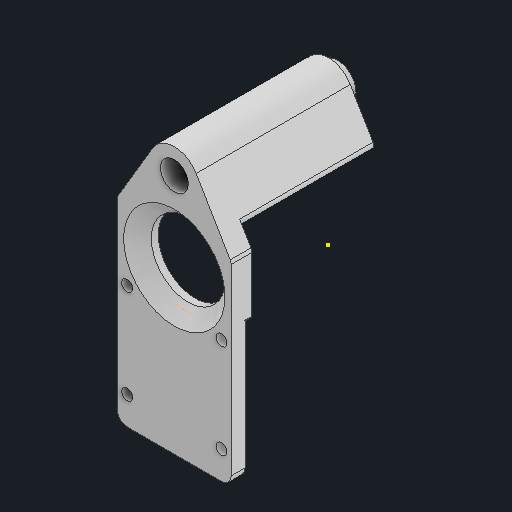
# Autodesk Inventor part: servo_side_plate1
Saved by Autodesk Inventor 2026 (Build 300175000, 175)
## iProperties
Created: 2025-12-05
Part Number: servo_side_plate1
Material: Generic
Document SubType Name: Modeling
Designer: numai
Density: 1 g/cm^3
Appearance: Default
Author: numai
Autodesk Inventor part; units mm, degrees
ref_plane "YZ Plane" through (0, 0, 0) normal (1, 0, 0) x (0, 1, 0)
ref_plane "XZ Plane" through (0, 0, 0) normal (0, 1, 0) x (-1, 0, 0)
ref_plane "XY Plane" through (0, 0, 0) normal (0, 0, 1) x (1, 0, 0)
ref_plane "作業平面1" through (0, -9.5185, 2.5) normal (0, 0, 1) x (1, 0, 0)
sketch "スケッチ1" plane through (0, -9.5185, 2.5) normal (0, 0, 1) x (1, 0, 0)
  arc A0 (6.111, 12.2244) -> (9.9756, 16.2085) centre (0, 22.0185) ccw construction
  arc A1 (7, 11.2305) -> (6.111, 12.2244) centre (6, 11.2305) ccw construction
  line L0 (7, 11.2305) -> (7, -12.0915) construction
  arc A2 (6.6057, -12.8872) -> (7, -12.0915) centre (6, -12.0915) ccw construction
  arc A3 (6.6057, -12.8872) -> (7.8, -11.5915) centre (6.5, -11.5915) ccw construction
  line L1 (7.8, -10.5915) -> (7.8, -11.5915) construction
  arc A4 (10.11, -8.2815) -> (7.8, -10.5915) centre (10.11, -10.5915) ccw construction
  line L2 (10.86, -8.2815) -> (10.11, -8.2815) construction
  arc A5 (10.86, -8.2815) -> (12.16, -6.9815) centre (10.86, -6.9815) ccw construction
  line L3 (12.16, 16.2085) -> (12.16, -6.9815) construction
  line L4 (9.9756, 16.2085) -> (12.16, 16.2085) construction
  circle A6 centre (10.25, 13.5185) radius 0.7835 construction
  circle A7 centre (10.25, -6.9815) radius 0.7835 construction
  arc A8 (-7.8, -11.5915) -> (-6.6057, -12.8872) centre (-6.5, -11.5915) ccw construction
  arc A9 (-7, -12.0915) -> (-6.6057, -12.8872) centre (-6, -12.0915) ccw construction
  line L5 (-7, -12.0915) -> (-7, 11.2305) construction
  arc A10 (-6.111, 12.2244) -> (-7, 11.2305) centre (-6, 11.2305) ccw construction
  arc A11 (-9.9756, 16.2085) -> (-6.111, 12.2244) centre (0, 22.0185) ccw construction
  line L6 (-12.16, 16.2085) -> (-9.9756, 16.2085) construction
  line L7 (-12.16, -6.9815) -> (-12.16, 16.2085) construction
  arc A12 (-12.16, -6.9815) -> (-10.86, -8.2815) centre (-10.86, -6.9815) ccw construction
  line L8 (-10.11, -8.2815) -> (-10.86, -8.2815) construction
  arc A13 (-7.8, -10.5915) -> (-10.11, -8.2815) centre (-10.11, -10.5915) ccw construction
  line L9 (-7.8, -11.5915) -> (-7.8, -10.5915) construction
  circle A14 centre (-10.25, 13.5185) radius 0.7835 construction
  circle A15 centre (-10.25, -6.9815) radius 0.7835 construction
  line L10 (-12.36, 16.2085) -> (-12.36, -6.9815) construction
  line L11 (12.36, -6.9815) -> (12.36, 16.2085) construction
  circle A16 centre (0, 22.0185) radius 3.4 construction
  arc A17 (5.25, 16.6624) -> (-5.25, 16.6624) centre (0, 22.0185) ccw construction
  arc A18 (-5.25, 16.6624) -> (5.25, 16.6624) centre (0, 22.0185) ccw construction
  circle A19 centre (0, 22.0185) radius 8
  arc A20 (10.25, -13.0915) -> (12.36, -10.9815) centre (10.25, -10.9815) ccw construction
  arc A21 (-12.36, -10.9815) -> (-10.25, -13.0915) centre (-10.25, -10.9815) ccw construction
  arc A22 (-11.9207, 29.8679) -> (-12.36, 28.8072) centre (-10.86, 28.8072) ccw projected
  line L12 (-10.0993, 31.6892) -> (-11.9207, 29.8679) projected
  arc A23 (-9.0387, 32.1285) -> (-10.0993, 31.6892) centre (-9.0387, 30.6285) ccw projected
  arc A24 (10.0993, 31.6892) -> (9.0387, 32.1285) centre (9.0387, 30.6285) ccw projected
  line L13 (11.9207, 29.8679) -> (10.0993, 31.6892) projected
  arc A25 (12.36, 28.8072) -> (11.9207, 29.8679) centre (10.86, 28.8072) ccw projected
  circle A26 centre (9.36, 29.1285) radius 0.7835 construction
  circle A27 centre (-9.36, 29.1285) radius 0.7835 construction
  line L14 (12.16, 16.4085) -> (9.9756, 16.4085) construction
  arc A28 (5.5139, 12.1045) -> (9.8028, 16.3092) centre (0, 22.0185) ccw construction
  arc A29 (-9.8028, 16.3092) -> (-5.5139, 12.1045) centre (0, 22.0185) ccw construction
  line L15 (-9.9756, 16.4085) -> (-12.16, 16.4085) construction
  line L16 (-12.36, 28.8072) -> (-12.36, 16.2085) projected
  line L17 (12.36, 16.2085) -> (12.36, 28.8072) projected
  line L18 (9.0387, 32.1285) -> (-9.0387, 32.1285) projected
  line L19 (12.36, 16.4085) -> (9.86, 16.4085)
  arc A30 (-9.86, 16.4085) -> (9.86, 16.4085) centre (0, 22.0185) ccw
  line L20 (-9.86, 16.4085) -> (-12.36, 16.4085)
  point P0 (0, 9.5185)
  dimension "d0" = 16
  constraints: 5 point on line, 4 end point, 2 centre point, 2 coincident, 2 point on circle, 1 concentric, 1 horizontal
  measures "d0" diameter of A19
extrude "押し出し1" add sketch "スケッチ1" against normal blind 2.5
sketch "スケッチ2" plane through (0, -9.5185, 2.5) normal (0, 0, 1) x (1, 0, 0)
  line L0 (-12.36, 28.8072) -> (-12.36, 16.4085) projected
  line L1 (-12.36, 16.4085) -> (-9.86, 16.4085) projected
  arc A0 (-9.86, 16.4085) -> (9.86, 16.4085) centre (0, 22.0185) ccw projected
  line L2 (9.86, 16.4085) -> (12.36, 16.4085) projected
  line L3 (12.36, 16.4085) -> (12.36, 28.8072) projected
  arc A1 (12.36, 28.8072) -> (11.9207, 29.8679) centre (10.86, 28.8072) ccw projected
  line L4 (11.9207, 29.8679) -> (10.0993, 31.6892) projected
  arc A2 (10.0993, 31.6892) -> (9.0387, 32.1285) centre (9.0387, 30.6285) ccw projected
  line L5 (9.0387, 32.1285) -> (-9.0387, 32.1285) projected
  arc A3 (-9.0387, 32.1285) -> (-10.0993, 31.6892) centre (-9.0387, 30.6285) ccw projected
  line L6 (-10.0993, 31.6892) -> (-11.9207, 29.8679) projected
  arc A4 (-11.9207, 29.8679) -> (-12.36, 28.8072) centre (-10.86, 28.8072) ccw projected
  circle A5 centre (0, 22.0185) radius 8 projected
  line L7 (12.36, -10.9815) -> (12.36, -6.9815) projected
  line L8 (12.36, -6.9815) -> (12.36, 16.2085) projected
  line L9 (12.36, 16.2085) -> (12.36, 28.8072) projected
  line L10 (7, -12.0915) -> (7, 11.2305) projected
  arc A6 (10.25, -13.0915) -> (12.36, -10.9815) centre (10.25, -10.9815) ccw projected
  line L11 (6.5, -13.0915) -> (10.25, -13.0915) projected
  line L12 (-10.25, -13.0915) -> (-6.5, -13.0915) projected
  arc A7 (-12.36, -10.9815) -> (-10.25, -13.0915) centre (-10.25, -10.9815) ccw projected
  line L13 (-12.36, -6.9815) -> (-12.36, -10.9815) projected
  line L14 (-12.36, 16.2085) -> (-12.36, -6.9815) projected
  circle A8 centre (10.25, 13.5185) radius 0.7835 construction
  circle A9 centre (10.25, -6.9815) radius 0.7835 construction
  circle A10 centre (-10.25, 13.5185) radius 0.7835 construction
  circle A11 centre (-10.25, -6.9815) radius 0.7835 construction
  line L15 (-12.36, 28.8072) -> (-12.36, 16.2085) projected
  line L16 (-7, 11.2305) -> (-7, -12.0915) projected
  line L17 (7, 11.2305) -> (7, 13.0915)
  line L18 (7, -12.0915) -> (7, -13.0915)
  line L19 (-7, 11.2305) -> (-7, 13.0915)
  line L20 (-7, -12.0915) -> (-7, -13.0915)
  circle A12 centre (10.25, 13.5185) radius 1.2
  circle A13 centre (10.25, -6.9815) radius 1.2
  circle A14 centre (-10.25, 13.5185) radius 1.2
  circle A15 centre (-10.25, -6.9815) radius 1.2
  point P0 (0, 9.5185)
  dimension "d3" = 2.4
  constraints: 8 end point, 4 centre point, 4 coincident, 4 point on line, 3 equal radius, 2 point on circle, 1 parallel, 1 vertical
  measures "d3" diameter of A12
extrude "押し出し2" add sketch "スケッチ2" against normal blind 1 contours L1 A0 L19 L16 L20 L12 A7 L13 L14 L15 | A0 L2 L9 L8 L7 A6 L11 L18 L10 L17
sketch "スケッチ3" plane through (0, -9.5185, 2.5) normal (0, 0, 1) x (1, 0, 0)
  circle A0 centre (-10.25, 13.5185) radius 1.2 projected
  circle A1 centre (-10.25, -6.9815) radius 1.2 projected
  circle A2 centre (10.25, 13.5185) radius 1.2 projected
  circle A3 centre (10.25, -6.9815) radius 1.2 projected
  line L0 (-12.36, 28.8072) -> (-12.36, -10.9815) projected
  arc A4 (-12.36, -10.9815) -> (-10.25, -13.0915) centre (-10.25, -10.9815) ccw projected
  line L1 (-10.25, -13.0915) -> (-7, -13.0915) projected
  line L2 (-7, -13.0915) -> (-7, 13.0915) projected
  arc A5 (-7, 13.0915) -> (7, 13.0915) centre (0, 22.0185) ccw projected
  line L3 (7, 13.0915) -> (7, -13.0915) projected
  line L4 (7, -13.0915) -> (10.25, -13.0915) projected
  arc A6 (10.25, -13.0915) -> (12.36, -10.9815) centre (10.25, -10.9815) ccw projected
  line L5 (12.36, -10.9815) -> (12.36, 28.8072) projected
  arc A7 (12.36, 28.8072) -> (11.9207, 29.8679) centre (10.86, 28.8072) ccw projected
  line L6 (11.9207, 29.8679) -> (10.0993, 31.6892) projected
  arc A8 (10.0993, 31.6892) -> (9.0387, 32.1285) centre (9.0387, 30.6285) ccw projected
  line L7 (9.0387, 32.1285) -> (-9.0387, 32.1285) projected
  arc A9 (-9.0387, 32.1285) -> (-10.0993, 31.6892) centre (-9.0387, 30.6285) ccw projected
  line L8 (-10.0993, 31.6892) -> (-11.9207, 29.8679) projected
  arc A10 (-11.9207, 29.8679) -> (-12.36, 28.8072) centre (-10.86, 28.8072) ccw projected
  circle A11 centre (0, 22.0185) radius 8 projected
  line L9 (7, -13.0915) -> (-7, -13.0915)
  point P0 (0, 9.5185)
  constraints: 2 end point, 1 collinear
extrude "押し出し3" add sketch "スケッチ3" along normal blind 2
sketch "スケッチ4" plane through (0, -9.5185, 4.5) normal (0, 0, 1) x (1, 0, 0)
  arc A0 (10.25, -13.0915) -> (12.36, -10.9815) centre (10.25, -10.9815) ccw projected
  line L0 (12.36, -10.9815) -> (12.36, 28.8072) projected
  arc A1 (12.36, 28.8072) -> (11.9207, 29.8679) centre (10.86, 28.8072) ccw projected
  line L1 (11.9207, 29.8679) -> (10.0993, 31.6892) projected
  arc A2 (10.0993, 31.6892) -> (9.0387, 32.1285) centre (9.0387, 30.6285) ccw projected
  line L2 (9.0387, 32.1285) -> (-9.0387, 32.1285) projected
  arc A3 (-9.0387, 32.1285) -> (-10.0993, 31.6892) centre (-9.0387, 30.6285) ccw projected
  line L3 (-10.0993, 31.6892) -> (-11.9207, 29.8679) projected
  arc A4 (-11.9207, 29.8679) -> (-12.36, 28.8072) centre (-10.86, 28.8072) ccw projected
  line L4 (-12.36, 28.8072) -> (-12.36, -10.9815) projected
  arc A5 (-12.36, -10.9815) -> (-10.25, -13.0915) centre (-10.25, -10.9815) ccw projected
  line L5 (-10.25, -13.0915) -> (10.25, -13.0915) projected
  circle A6 centre (-10.25, 13.5185) radius 1.2 projected
  circle A7 centre (-10.25, -6.9815) radius 1.2 projected
  circle A8 centre (10.25, 13.5185) radius 1.2 projected
  circle A9 centre (10.25, -6.9815) radius 1.2 projected
  circle A10 centre (0, 22.0185) radius 8 projected
  line L6 (0, 22.0185) -> (0, 39.3185) construction
  circle A11 centre (0, 39.3185) radius 1.5
  circle A12 centre (0, 39.3185) radius 5.5 construction
  line L7 (-12.1513, 29.5705) -> (-4.7347, 42.1173)
  line L8 (12.1513, 29.5705) -> (4.7347, 42.1173)
  arc A13 (12.36, 28.8072) -> (11.9207, 29.8679) centre (10.86, 28.8072) ccw projected
  arc A14 (4.7347, 42.1173) -> (-4.7347, 42.1173) centre (0, 39.3185) ccw
  point P0 (0, 9.5185)
  dimension "d8" = 17.3
  dimension "d9" = 3
  dimension "d10" = 11
  constraints: 6 end point, 6 point on circle, 5 tangent, 3 centre point, 3 coincident, 1 vertical
  measures "d8" distance of L6.start L6.end
  measures "d9" diameter of A11
  measures "d10" diameter of A12
extrude "押し出し4" add sketch "スケッチ4" against normal up to surface (4.5 mm away) contours A1 L1 A2 L2 A3 L3 A4 L7 A14 L8
sketch "スケッチ5" plane through (0, -9.5185, 0) normal (0, 0, -1) x (-1, 0, 0)
  circle A0 centre (0, 39.3185) radius 1.5 projected
  line L0 (12.36, 16.4085) -> (12.36, 28.8072) projected
  arc A1 (12.36, 28.8072) -> (12.1513, 29.5705) centre (10.86, 28.8072) ccw projected
  line L1 (12.1513, 29.5705) -> (4.7347, 42.1173) projected
  arc A2 (4.7347, 42.1173) -> (-4.7347, 42.1173) centre (0, 39.3185) ccw projected
  line L2 (-4.7347, 42.1173) -> (-12.1513, 29.5705) projected
  arc A3 (-12.1513, 29.5705) -> (-12.36, 28.8072) centre (-10.86, 28.8072) ccw projected
  line L3 (-12.36, 28.8072) -> (-12.36, 16.4085) projected
  line L4 (-12.36, 16.4085) -> (-9.86, 16.4085) projected
  arc A4 (-9.86, 16.4085) -> (9.86, 16.4085) centre (0, 22.0185) ccw projected
  line L5 (9.86, 16.4085) -> (12.36, 16.4085) projected
  circle A5 centre (0, 22.0185) radius 8 projected
  arc A6 (-11.9207, 29.8679) -> (-12.36, 28.8072) centre (-10.86, 28.8072) ccw projected
  line L6 (-10.0993, 31.6892) -> (-11.9207, 29.8679) projected
  arc A7 (-9.0387, 32.1285) -> (-10.0993, 31.6892) centre (-9.0387, 30.6285) ccw projected
  line L7 (-0.95, 32.1285) -> (-9.0387, 32.1285) projected
  arc A8 (10.0993, 31.6892) -> (9.0387, 32.1285) centre (9.0387, 30.6285) ccw projected
  line L8 (11.9207, 29.8679) -> (10.0993, 31.6892) projected
  arc A9 (12.36, 28.8072) -> (11.9207, 29.8679) centre (10.86, 28.8072) ccw projected
  line L9 (9.0387, 32.1285) -> (0.95, 32.1285) projected
  line L10 (0.95, 32.1285) -> (-0.95, 32.1285) projected
  point P0 (0, 9.5185)
extrude "押し出し5" add sketch "スケッチ5" along normal blind 29 contours A9 L8 A8 L9 L10 L7 A7 L6 A6 L2 A2 L1
fillet "フィレット2" radius 0.4 4 edges at (7, -22.61, 2) (-7, -22.61, 2) (12.36, 6.89, 0.75) (-12.36, 6.89, 0.75)
sketch "スケッチ6" plane through (0, -9.5185, -29) normal (0, 0, -1) x (-1, 0, 0)
  circle A0 centre (0, 39.3185) radius 1.5 projected
  circle A1 centre (0, 39.3185) radius 4
  point P0 (0, 9.5185)
  dimension "d17" = 8
  constraints: 1 centre point, 1 coincident
  measures "d17" diameter of A1
extrude "押し出し6" add sketch "スケッチ6" along normal blind 2
sketch "スケッチ7" plane through (0, -9.5185, 2.5) normal (0, 0, -1) x (-1, 0, 0)
  line L0 (-7, 13.0915) -> (-7, -12.6915) projected
  arc A0 (-7.4, -13.0915) -> (-7, -12.6915) centre (-7.4, -12.6915) ccw projected
  line L1 (7.4, -13.0915) -> (-7.4, -13.0915) projected
  arc A1 (7, -12.6915) -> (7.4, -13.0915) centre (7.4, -12.6915) ccw projected
  line L2 (7, -12.6915) -> (7, 13.0915) projected
  arc A2 (-7, 13.0915) -> (7, 13.0915) centre (0, 22.0185) ccw projected
  line L3 (-7.1, -13.1915) -> (-7.1, 13.2994)
  arc A3 (-7.1, 13.2994) -> (7.1, 13.2994) centre (0, 22.0185) ccw
  line L4 (7.1, 13.2994) -> (7.1, -13.1915)
  line L5 (7.1, -13.1915) -> (-7.1, -13.1915)
  point P0 (0, 9.5185)
  point P1 (7.1, -12.9561)
  point P2 (-7.1, -12.9561)
  point P3 (7.1, -13.0915)
  point P4 (-7.1, -13.0915)
  dimension "d20" = 0.1
  constraints: 6 end point, 2 point on circle, 1 centre point, 3 other
  measures "d20" distance between parallel lines of L5 L1
extrude "押し出し7" cut sketch "スケッチ7" along normal through all contours L0 A0 L3 A3 L4 A1 L2 A2 | L1 L4 L5 L3
sketch "スケッチ8" plane through (0, -9.5185, 1.5) normal (0, 0, -1) x (-1, 0, 0)
  line L0 (-7.1, -12.9561) -> (-7.1, 13.1708) projected
  arc A0 (-9.86, 16.4085) -> (-7.1, 13.1708) centre (0, 22.0185) ccw projected
  line L1 (-11.96, 16.4085) -> (-9.86, 16.4085) projected
  arc A1 (-12.36, 16.8085) -> (-11.96, 16.4085) centre (-11.96, 16.8085) ccw projected
  line L2 (-12.36, 16.8085) -> (-12.36, -10.9815) projected
  arc A2 (-12.36, -10.9815) -> (-10.25, -13.0915) centre (-10.25, -10.9815) ccw projected
  line L3 (-10.25, -13.0915) -> (-7.4, -13.0915) projected
  arc A3 (-7.4, -13.0915) -> (-7.1, -12.9561) centre (-7.4, -12.6915) ccw projected
  circle A4 centre (-10.25, -6.9815) radius 1.2 projected
  circle A5 centre (-10.25, 13.5185) radius 1.2 projected
  circle A6 centre (10.25, 13.5185) radius 1.2 projected
  circle A7 centre (10.25, -6.9815) radius 1.2 projected
  line L4 (7.1, 13.1708) -> (7.1, -12.9561) projected
  arc A8 (7.1, -12.9561) -> (7.4, -13.0915) centre (7.4, -12.6915) ccw projected
  line L5 (7.4, -13.0915) -> (10.25, -13.0915) projected
  arc A9 (10.25, -13.0915) -> (12.36, -10.9815) centre (10.25, -10.9815) ccw projected
  line L6 (12.36, -10.9815) -> (12.36, 16.8085) projected
  arc A10 (11.96, 16.4085) -> (12.36, 16.8085) centre (11.96, 16.8085) ccw projected
  line L7 (9.86, 16.4085) -> (11.96, 16.4085) projected
  arc A11 (7.1, 13.1708) -> (9.86, 16.4085) centre (0, 22.0185) ccw projected
  line L8 (-12.46, -10.9815) -> (-12.46, 16.5085)
  line L9 (-12.46, 16.5085) -> (-9.8017, 16.5085)
  arc A12 (-9.8017, 16.5085) -> (-7, 13.2189) centre (0, 22.0185) ccw
  line L10 (-7, 13.2189) -> (-7, -12.9915)
  arc A13 (-7.4, -13.1915) -> (-7, -12.9915) centre (-7.4, -12.6915) ccw
  line L11 (-7.4, -13.1915) -> (-10.25, -13.1915)
  arc A14 (-12.46, -10.9815) -> (-10.25, -13.1915) centre (-10.25, -10.9815) ccw
  line L12 (12.46, 16.5085) -> (12.46, -10.9815)
  arc A15 (10.25, -13.1915) -> (12.46, -10.9815) centre (10.25, -10.9815) ccw
  line L13 (10.25, -13.1915) -> (7.4, -13.1915)
  arc A16 (7, -12.9915) -> (7.4, -13.1915) centre (7.4, -12.6915) ccw
  line L14 (7, -12.9915) -> (7, 13.2189)
  arc A17 (7, 13.2189) -> (9.8017, 16.5085) centre (0, 22.0185) ccw
  line L15 (9.8017, 16.5085) -> (12.46, 16.5085)
  point P0 (0, 9.5185)
  point P1 (-12.36, 16.5085)
  point P2 (-12.2246, 16.5085)
  point P3 (12.2246, 16.5085)
  point P4 (12.36, 16.5085)
  dimension "d23" = 0.1
  dimension "d24" = 0.1
  constraints: 16 end point, 12 point on circle, 6 centre point, 12 other
  measures "d23" distance between parallel lines of L8 L2
  measures "d24" distance between parallel lines of L12 L6
extrude "押し出し8" cut sketch "スケッチ8" along normal through all contours L0 A0 L1 A1 L9 A12 L10 A13 L11 A14 L8 L2 A2 L3 A3 | L4 A8 L5 A9 L6 L15 L12 A15 L13 A16 L14 A17 A10 L7 A11
chamfer "面取り1" distance 3 angle 45 1 edges at (-8, 12.5, 4.5)
sketch "スケッチ9" plane through (0, -9.5185, -29) normal (0, 0, -1) x (-1, 0, 0)
  point P0 (0, 9.5185)
sketch "スケッチ10" plane through (0, -9.5185, -29) normal (0, 0, -1) x (-1, 0, 0)
  circle A0 centre (0, 22.0185) radius 8 projected
  line L0 (-12.2246, 16.5085) -> (-9.8017, 16.5085) projected
  arc A1 (-9.8017, 16.5085) -> (9.8017, 16.5085) centre (0, 22.0185) ccw projected
  line L1 (9.8017, 16.5085) -> (12.2246, 16.5085) projected
  arc A2 (12.2246, 16.5085) -> (12.36, 16.8085) centre (11.96, 16.8085) ccw projected
  line L2 (12.36, 16.8085) -> (12.36, 28.8072) projected
  arc A3 (12.36, 28.8072) -> (12.1513, 29.5705) centre (10.86, 28.8072) ccw projected
  arc A4 (12.1513, 29.5705) -> (11.9207, 29.8679) centre (10.86, 28.8072) ccw projected
  line L3 (11.9207, 29.8679) -> (10.0993, 31.6892) projected
  arc A5 (10.0993, 31.6892) -> (9.0387, 32.1285) centre (9.0387, 30.6285) ccw projected
  line L4 (9.0387, 32.1285) -> (-9.0387, 32.1285) projected
  arc A6 (-9.0387, 32.1285) -> (-10.0993, 31.6892) centre (-9.0387, 30.6285) ccw projected
  line L5 (-10.0993, 31.6892) -> (-11.9207, 29.8679) projected
  arc A7 (-11.9207, 29.8679) -> (-12.1513, 29.5705) centre (-10.86, 28.8072) ccw projected
  arc A8 (-12.1513, 29.5705) -> (-12.36, 28.8072) centre (-10.86, 28.8072) ccw projected
  line L6 (-12.36, 28.8072) -> (-12.36, 16.8085) projected
  arc A9 (-12.36, 16.8085) -> (-12.2246, 16.5085) centre (-11.96, 16.8085) ccw projected
  line L7 (-9.0387, 32.2285) -> (9.0387, 32.2285)
  arc A10 (10.1701, 31.7599) -> (9.0387, 32.2285) centre (9.0387, 30.6285) ccw
  line L8 (10.1701, 31.7599) -> (11.9914, 29.9386)
  arc A11 (12.2286, 29.636) -> (11.9914, 29.9386) centre (10.86, 28.8072) ccw
  arc A12 (12.46, 28.8072) -> (12.2286, 29.636) centre (10.86, 28.8072) ccw
  line L9 (12.46, 28.8072) -> (12.46, 16.8085)
  arc A13 (12.26, 16.4085) -> (12.46, 16.8085) centre (11.96, 16.8085) ccw
  line L10 (12.26, 16.4085) -> (9.86, 16.4085)
  arc A14 (-9.86, 16.4085) -> (9.86, 16.4085) centre (0, 22.0185) ccw
  line L11 (-9.86, 16.4085) -> (-12.26, 16.4085)
  arc A15 (-12.46, 16.8085) -> (-12.26, 16.4085) centre (-11.96, 16.8085) ccw
  line L12 (-12.46, 16.8085) -> (-12.46, 28.8072)
  arc A16 (-12.2286, 29.636) -> (-12.46, 28.8072) centre (-10.86, 28.8072) ccw
  arc A17 (-11.9914, 29.9386) -> (-12.2286, 29.636) centre (-10.86, 28.8072) ccw
  line L13 (-11.9914, 29.9386) -> (-10.1701, 31.7599)
  arc A18 (-9.0387, 32.2285) -> (-10.1701, 31.7599) centre (-9.0387, 30.6285) ccw
  point P0 (0, 9.5185)
  dimension "d30" = 0.1
  constraints: 18 point on circle, 14 end point, 9 centre point, 15 other
  measures "d30" distance between parallel lines of L4 L7
extrude "押し出し9" cut sketch "スケッチ10" against normal up to surface (29 mm away) contours A0 | A9 L6 A8 A7 L5 A6 L4 A5 L3 A4 A3 L2 A2 L1 A1 L0 | L7 A10 L8 A11 A12 L9 A13 L10 A14 L11 A15 L12 A16 A17 L13 A18
fillet "フィレット3" radius 1 2 edges at (11.8503, 20.5611, -14.5) (-11.8503, 20.5611, -14.5)
sketch "スケッチ11" plane through (0, -9.5185, 4.5) normal (0, 0, 1) x (1, 0, 0)
  circle A0 centre (0, 39.3185) radius 1.5 construction
  circle A1 centre (0, 39.3185) radius 3.05
  point P0 (0, 9.5185)
  dimension "d34" = 6.1
  constraints: 1 centre point, 1 coincident
  measures "d34" diameter of A1
extrude "押し出し10" cut sketch "スケッチ11" against normal through all
equation "\"d24\" = d23"
